Autodesk Fusion 360 part; units mm, degrees
note: some values were not read from the file. Set by a fixed rule: which face or edge a step refers to.
(part 3 of 12)
  spline S7 degree 5 poles (4.6371, -4.3427) (4.637, -4.3399) (4.6367, -4.3344) (4.6362, -4.326) (4.6355, -4.3149) (4.6346, -4.3011) (4.6336, -4.2873) (4.6327, -4.2735) (4.6316, -4.2598) (4.6306, -4.2461) (4.6295, -4.2324) (4.6283, -4.2188) (4.6271, -4.2052) (4.6259, -4.1917) (4.6246, -4.1782) (4.6233, -4.1647) (4.622, -4.1512) (4.6206, -4.1378) (4.6192, -4.1244) (4.6177, -4.1111) (4.6162, -4.0978) (4.6146, -4.0846) (4.6131, -4.0713) (4.6114, -4.0582) (4.6098, -4.045) (4.6081, -4.0319) (4.6063, -4.0188) (4.6045, -4.0058) (4.6027, -3.9928) (4.6009, -3.9799) (4.599, -3.967) (4.597, -3.9541) (4.5951, -3.9413) (4.5931, -3.9285) (4.591, -3.9157) (4.589, -3.903) (4.5868, -3.8904) (4.5847, -3.8778) (4.5825, -3.8652) (4.5803, -3.8526) (4.578, -3.8401) (4.5757, -3.8277) (4.5734, -3.8153) (4.5711, -3.8029) (4.5687, -3.7906) (4.5662, -3.7783) (4.5638, -3.766) (4.5613, -3.7538) (4.5587, -3.7417) (4.5562, -3.7296) (4.5536, -3.7175) (4.5509, -3.7055) (4.5483, -3.6935) (4.5456, -3.6816) (4.5429, -3.6697) (4.5401, -3.6578) (4.5373, -3.646) (4.5345, -3.6343) (4.5316, -3.6226) (4.5287, -3.6109) (4.5258, -3.5993) (4.5229, -3.5877) (4.5199, -3.5762) (4.5169, -3.5647) (4.5139, -3.5533) (4.5108, -3.5419) (4.5077, -3.5306) (4.5046, -3.5193) (4.5014, -3.508) (4.4983, -3.4969) (4.495, -3.4857) (4.4918, -3.4746) (4.4886, -3.4636) (4.4853, -3.4526) (4.4819, -3.4416) (4.4786, -3.4307) (4.4752, -3.4199) (4.4718, -3.4091) (4.4684, -3.3983) (4.465, -3.3876) (4.4615, -3.377) (4.458, -3.3664) (4.4545, -3.3558) (4.4509, -3.3453) (4.4474, -3.3349) (4.4438, -3.3245) (4.4402, -3.3141) (4.4365, -3.3039) (4.4329, -3.2936) (4.4292, -3.2834) (4.4255, -3.2733) (4.4218, -3.2632) (4.418, -3.2532) (4.4143, -3.2432) (4.4105, -3.2333) (4.4067, -3.2234) (4.4028, -3.2136) (4.399, -3.2038) (4.3951, -3.1941) (4.3912, -3.1845) (4.3873, -3.1749) (4.3834, -3.1653) (4.3795, -3.1558) (4.3755, -3.1464) (4.3715, -3.137) (4.3676, -3.1277) (4.3635, -3.1184) (4.3595, -3.1092) (4.3555, -3.1) (4.3514, -3.0909) (4.3474, -3.0819) (4.3433, -3.0729) (4.3392, -3.064) (4.3351, -3.0551) (4.331, -3.0463) (4.3268, -3.0375) (4.3227, -3.0288) (4.3185, -3.0202) (4.3143, -3.0116) (4.3102, -3.003) (4.306, -2.9946) (4.3018, -2.9862) (4.2975, -2.9778) (4.2933, -2.9695) (4.2891, -2.9613) (4.2848, -2.9531) (4.2806, -2.945) (4.2763, -2.9369) (4.2721, -2.9289) (4.2678, -2.921) (4.2635, -2.9131) (4.2592, -2.9053) (4.2549, -2.8975) (4.2507, -2.8898) (4.2464, -2.8822) (4.2421, -2.8746) (4.2377, -2.8671) (4.2334, -2.8596) (4.2291, -2.8522) (4.2248, -2.8449) (4.2205, -2.8376) (4.2162, -2.8304) (4.2119, -2.8233) (4.2075, -2.8162) (4.2032, -2.8092) (4.1989, -2.8022) (4.1946, -2.7953) (4.1903, -2.7885) (4.186, -2.7817) (4.1817, -2.775) (4.1774, -2.7684) (4.1731, -2.7618) (4.1688, -2.7553) (4.1645, -2.7488) (4.1602, -2.7424) (4.1559, -2.7361) (4.1516, -2.7298) (4.1474, -2.7236) (4.1431, -2.7175) (4.1389, -2.7115) (4.1346, -2.7055) (4.1304, -2.6995) (4.1262, -2.6936) (4.122, -2.6878) (4.1178, -2.6821) (4.1136, -2.6764) (4.1095, -2.6708) (4.1053, -2.6653) (4.1012, -2.6598) (4.097, -2.6544) (4.0929, -2.6491) (4.0888, -2.6438) (4.0848, -2.6386) (4.0807, -2.6335) (4.0767, -2.6284) (4.0726, -2.6234) (4.0686, -2.6184) (4.0647, -2.6136) (4.0607, -2.6088) (4.0568, -2.604) (4.0529, -2.5994) (4.049, -2.5948) (4.0451, -2.5902) (4.0413, -2.5858) (4.0375, -2.5814) (4.0337, -2.577) (4.0299, -2.5728) (4.0262, -2.5686) (4.0225, -2.5645) (4.0188, -2.5604) (4.0152, -2.5565) (4.0116, -2.5525) (4.008, -2.5487) (4.0044, -2.5449) (4.0009, -2.5412) (3.9975, -2.5376) (3.994, -2.534) (3.9906, -2.5305) (3.9873, -2.5271) (3.9839, -2.5237) (3.9807, -2.5205) (3.9774, -2.5172) (3.9742, -2.5141) (3.9711, -2.511) (3.968, -2.508) (3.9649, -2.5051) (3.9619, -2.5022) (3.9589, -2.4994) (3.956, -2.4967) (3.9531, -2.4941) (3.9503, -2.4915) (3.9475, -2.489) (3.9448, -2.4865) (3.9421, -2.4842) (3.9395, -2.4819) (3.937, -2.4797) (3.9345, -2.4775) (3.9321, -2.4754) (3.9297, -2.4734) (3.9274, -2.4715) (3.9251, -2.4696) (3.9229, -2.4678) (3.9208, -2.4661) (3.9188, -2.4644) (3.9168, -2.4629) (3.9149, -2.4613) (3.9131, -2.4599) (3.9113, -2.4585) (3.9096, -2.4572) (3.908, -2.456) (3.9065, -2.4549) (3.905, -2.4538) (3.9036, -2.4528) (3.9023, -2.4518) (3.9011, -2.451) (3.9, -2.4502) (3.899, -2.4495) (3.8981, -2.4488) (3.8972, -2.4482) (3.8965, -2.4477) (3.8958, -2.4473) (3.8954, -2.447) (3.8951, -2.4468) (3.8949, -2.4467) (3.8949, -2.4466) knots -1 -1 -1 -1 -1 -1 -0.99583333 -0.99166667 -0.9875 -0.98333333 -0.97916667 -0.975 -0.97083333 -0.96666667 -0.9625 -0.95833333 -0.95416667 -0.95 -0.94583333 -0.94166667 -0.9375 -0.93333333 -0.92916667 -0.925 -0.92083333 -0.91666667 -0.9125 -0.90833333 -0.90416667 -0.9 -0.89583333 -0.89166667 -0.8875 -0.88333333 -0.87916667 -0.875 -0.87083333 -0.86666667 -0.8625 -0.85833333 -0.85416667 -0.85 -0.84583333 -0.84166667 -0.8375 -0.83333333 -0.82916667 -0.825 -0.82083333 -0.81666667 -0.8125 -0.80833333 -0.80416667 -0.8 -0.79583333 -0.79166667 -0.7875 -0.78333333 -0.77916667 -0.775 -0.77083333 -0.76666667 -0.7625 -0.75833333 -0.75416667 -0.75 -0.74583333 -0.74166667 -0.7375 -0.73333333 -0.72916667 -0.725 -0.72083333 -0.71666667 -0.7125 -0.70833333 -0.70416667 -0.7 -0.69583333 -0.69166667 -0.6875 -0.68333333 -0.67916667 -0.675 -0.67083333 -0.66666667 -0.6625 -0.65833333 -0.65416667 -0.65 -0.64583333 -0.64166667 -0.6375 -0.63333333 -0.62916667 -0.625 -0.62083333 -0.61666667 -0.6125 -0.60833333 -0.60416667 -0.6 -0.59583333 -0.59166667 -0.5875 -0.58333333 -0.57916667 -0.575 -0.57083333 -0.56666667 -0.5625 -0.55833333 -0.55416667 -0.55 -0.54583333 -0.54166667 -0.5375 -0.53333333 -0.52916667 -0.525 -0.52083333 -0.51666667 -0.5125 -0.50833333 -0.50416667 -0.5 -0.49583333 -0.49166667 -0.4875 -0.48333333 -0.47916667 -0.475 -0.47083333 -0.46666667 -0.4625 -0.45833333 -0.45416667 -0.45 -0.44583333 -0.44166667 -0.4375 -0.43333333 -0.42916667 -0.425 -0.42083333 -0.41666667 -0.4125 -0.40833333 -0.40416667 -0.4 -0.39583333 -0.39166667 -0.3875 -0.38333333 -0.37916667 -0.375 -0.37083333 -0.36666667 -0.3625 -0.35833333 -0.35416667 -0.35 -0.34583333 -0.34166667 -0.3375 -0.33333333 -0.32916667 -0.325 -0.32083333 -0.31666667 -0.3125 -0.30833333 -0.30416667 -0.3 -0.29583333 -0.29166667 -0.2875 -0.28333333 -0.27916667 -0.275 -0.27083333 -0.26666667 -0.2625 -0.25833333 -0.25416667 -0.25 -0.24583333 -0.24166667 -0.2375 -0.23333333 -0.22916667 -0.225 -0.22083333 -0.21666667 -0.2125 -0.20833333 -0.20416667 -0.2 -0.19583333 -0.19166667 -0.1875 -0.18333333 -0.17916667 -0.175 -0.17083333 -0.16666667 -0.1625 -0.15833333 -0.15416667 -0.15 -0.14583333 -0.14166667 -0.1375 -0.13333333 -0.12916667 -0.125 -0.12083333 -0.11666667 -0.1125 -0.10833333 -0.10416667 -0.1 -0.09583333 -0.09166667 -0.0875 -0.08333333 -0.07916667 -0.075 -0.07083333 -0.06666667 -0.0625 -0.05833333 -0.05416667 -0.05 -0.04583333 -0.04166667 -0.0375 -0.03333333 -0.02916667 -0.025 -0.02083333 -0.01666667 -0.0125 -0.00833333 -0.00416667 0 0 0 0 0 0
  line L14 (3.8949, -2.4466) -> (3.8941, -2.4462)
  line L15 (3.8941, -2.4462) -> (3.1172, -1.9582)
  arc A8 (3.1172, -1.9582) -> (3.5889, -0.8196) centre (0, 0) ccw
  line L16 (3.5889, -0.8196) -> (4.4833, -1.0239)
  line L17 (4.4833, -1.0239) -> (4.4841, -1.024)
  spline S8 degree 5 poles (4.4841, -1.024) (4.4842, -1.0241) (4.4844, -1.0241) (4.4848, -1.0242) (4.4853, -1.0243) (4.486, -1.0244) (4.4869, -1.0246) (4.4879, -1.0248) (4.489, -1.025) (4.4903, -1.0252) (4.4916, -1.0254) (4.4931, -1.0257) (4.4947, -1.0259) (4.4963, -1.0262) (4.4981, -1.0264) (4.5, -1.0267) (4.502, -1.027) (4.5042, -1.0272) (4.5064, -1.0275) (4.5087, -1.0278) (4.5111, -1.0281) (4.5136, -1.0284) (4.5162, -1.0287) (4.5189, -1.0289) (4.5218, -1.0292) (4.5247, -1.0295) (4.5277, -1.0297) (4.5308, -1.03) (4.534, -1.0302) (4.5372, -1.0305) (4.5406, -1.0307) (4.5441, -1.0309) (4.5476, -1.0311) (4.5513, -1.0313) (4.555, -1.0315) (4.5588, -1.0317) (4.5627, -1.0319) (4.5667, -1.032) (4.5708, -1.0321) (4.575, -1.0322) (4.5792, -1.0323) (4.5835, -1.0324) (4.5879, -1.0325) (4.5924, -1.0325) (4.597, -1.0325) (4.6016, -1.0325) (4.6064, -1.0325) (4.6111, -1.0324) (4.616, -1.0324) (4.621, -1.0323) (4.626, -1.0322) (4.6311, -1.032) (4.6363, -1.0319) (4.6415, -1.0317) (4.6468, -1.0315) (4.6522, -1.0312) (4.6577, -1.031) (4.6632, -1.0307) (4.6688, -1.0303) (4.6745, -1.03) (4.6802, -1.0296) (4.686, -1.0292) (4.6919, -1.0288) (4.6978, -1.0283) (4.7038, -1.0278) (4.7099, -1.0272) (4.716, -1.0267) (4.7222, -1.0261) (4.7285, -1.0255) (4.7348, -1.0248) (4.7412, -1.0241) (4.7476, -1.0234) (4.7541, -1.0226) (4.7607, -1.0218) (4.7673, -1.021) (4.774, -1.0201) (4.7807, -1.0192) (4.7875, -1.0182) (4.7944, -1.0173) (4.8013, -1.0162) (4.8083, -1.0152) (4.8153, -1.0141) (4.8224, -1.013) (4.8295, -1.0118) (4.8367, -1.0106) (4.8439, -1.0093) (4.8512, -1.0081) (4.8585, -1.0067) (4.8659, -1.0054) (4.8734, -1.004) (4.8809, -1.0025) (4.8884, -1.001) (4.896, -0.9995) (4.9037, -0.9979) (4.9114, -0.9963) (4.9191, -0.9947) (4.9269, -0.993) (4.9347, -0.9912) (4.9426, -0.9894) (4.9505, -0.9876) (4.9585, -0.9858) (4.9665, -0.9838) (4.9746, -0.9819) (4.9827, -0.9799) (4.9908, -0.9778) (4.999, -0.9757) (5.0073, -0.9736) (5.0155, -0.9714) (5.0239, -0.9692) (5.0322, -0.9669) (5.0406, -0.9646) (5.0491, -0.9623) (5.0576, -0.9599) (5.0661, -0.9574) (5.0746, -0.9549) (5.0832, -0.9524) (5.0919, -0.9498) (5.1005, -0.9471) (5.1092, -0.9444) (5.118, -0.9417) (5.1268, -0.9389) (5.1356, -0.9361) (5.1444, -0.9332) (5.1533, -0.9303) (5.1623, -0.9273) (5.1712, -0.9243) (5.1802, -0.9212) (5.1892, -0.9181) (5.1983, -0.9149) (5.2074, -0.9117) (5.2165, -0.9084) (5.2256, -0.9051) (5.2348, -0.9017) (5.244, -0.8983) (5.2533, -0.8948) (5.2626, -0.8913) (5.2719, -0.8877) (5.2812, -0.8841) (5.2905, -0.8804) (5.2999, -0.8767) (5.3094, -0.8729) (5.3188, -0.8691) (5.3283, -0.8652) (5.3378, -0.8613) (5.3473, -0.8573) (5.3568, -0.8533) (5.3664, -0.8492) (5.376, -0.8451) (5.3856, -0.8409) (5.3953, -0.8367) (5.4049, -0.8324) (5.4146, -0.8281) (5.4244, -0.8237) (5.4341, -0.8192) (5.4439, -0.8147) (5.4537, -0.8102) (5.4635, -0.8056) (5.4733, -0.8009) (5.4831, -0.7962) (5.493, -0.7915) (5.5029, -0.7867) (5.5128, -0.7818) (5.5227, -0.7769) (5.5327, -0.7719) (5.5426, -0.7669) (5.5526, -0.7618) (5.5626, -0.7567) (5.5726, -0.7515) (5.5827, -0.7463) (5.5927, -0.741) (5.6028, -0.7356) (5.6129, -0.7302) (5.623, -0.7248) (5.6331, -0.7193) (5.6432, -0.7137) (5.6534, -0.7081) (5.6636, -0.7024) (5.6737, -0.6967) (5.6839, -0.6909) (5.6941, -0.6851) (5.7043, -0.6792) (5.7146, -0.6733) (5.7248, -0.6673) (5.7351, -0.6613) (5.7453, -0.6552) (5.7556, -0.649) (5.7659, -0.6428) (5.7762, -0.6365) (5.7865, -0.6302) (5.7968, -0.6239) (5.8071, -0.6174) (5.8175, -0.611) (5.8278, -0.6044) (5.8382, -0.5978) (5.8485, -0.5912) (5.8589, -0.5845) (5.8693, -0.5777) (5.8797, -0.5709) (5.8901, -0.5641) (5.9005, -0.5572) (5.9109, -0.5502) (5.9213, -0.5432) (5.9317, -0.5361) (5.9421, -0.529) (5.9525, -0.5218) (5.963, -0.5145) (5.9734, -0.5072) (5.9839, -0.4999) (5.9943, -0.4925) (6.0048, -0.485) (6.0152, -0.4775) (6.0257, -0.4699) (6.0361, -0.4623) (6.0466, -0.4546) (6.057, -0.4469) (6.0675, -0.4391) (6.078, -0.4313) (6.0884, -0.4234) (6.0989, -0.4154) (6.1094, -0.4074) (6.1199, -0.3993) (6.1303, -0.3912) (6.1408, -0.383) (6.1513, -0.3748) (6.1617, -0.3665) (6.1722, -0.3582) (6.1827, -0.3498) (6.1931, -0.3414) (6.2036, -0.3329) (6.2141, -0.3243) (6.2245, -0.3157) (6.235, -0.3071) (6.2454, -0.2983) (6.2559, -0.2896) (6.2663, -0.2807) (6.2768, -0.2719) (6.2872, -0.2629) (6.2976, -0.2539) (6.3081, -0.2449) (6.3185, -0.2358) (6.3289, -0.2267) (6.3372, -0.2193) (6.3435, -0.2137) (6.3476, -0.21) (6.3497, -0.2082) knots 0 0 0 0 0 0 0.00416667 0.00833333 0.0125 0.01666667 0.02083333 0.025 0.02916667 0.03333333 0.0375 0.04166667 0.04583333 0.05 0.05416667 0.05833333 0.0625 0.06666667 0.07083333 0.075 0.07916667 0.08333333 0.0875 0.09166667 0.09583333 0.1 0.10416667 0.10833333 0.1125 0.11666667 0.12083333 0.125 0.12916667 0.13333333 0.1375 0.14166667 0.14583333 0.15 0.15416667 0.15833333 0.1625 0.16666667 0.17083333 0.175 0.17916667 0.18333333 0.1875 0.19166667 0.19583333 0.2 0.20416667 0.20833333 0.2125 0.21666667 0.22083333 0.225 0.22916667 0.23333333 0.2375 0.24166667 0.24583333 0.25 0.25416667 0.25833333 0.2625 0.26666667 0.27083333 0.275 0.27916667 0.28333333 0.2875 0.29166667 0.29583333 0.3 0.30416667 0.30833333 0.3125 0.31666667 0.32083333 0.325 0.32916667 0.33333333 0.3375 0.34166667 0.34583333 0.35 0.35416667 0.35833333 0.3625 0.36666667 0.37083333 0.375 0.37916667 0.38333333 0.3875 0.39166667 0.39583333 0.4 0.40416667 0.40833333 0.4125 0.41666667 0.42083333 0.425 0.42916667 0.43333333 0.4375 0.44166667 0.44583333 0.45 0.45416667 0.45833333 0.4625 0.46666667 0.47083333 0.475 0.47916667 0.48333333 0.4875 0.49166667 0.49583333 0.5 0.50416667 0.50833333 0.5125 0.51666667 0.52083333 0.525 0.52916667 0.53333333 0.5375 0.54166667 0.54583333 0.55 0.55416667 0.55833333 0.5625 0.56666667 0.57083333 0.575 0.57916667 0.58333333 0.5875 0.59166667 0.59583333 0.6 0.60416667 0.60833333 0.6125 0.61666667 0.62083333 0.625 0.62916667 0.63333333 0.6375 0.64166667 0.64583333 0.65 0.65416667 0.65833333 0.6625 0.66666667 0.67083333 0.675 0.67916667 0.68333333 0.6875 0.69166667 0.69583333 0.7 0.70416667 0.70833333 0.7125 0.71666667 0.72083333 0.725 0.72916667 0.73333333 0.7375 0.74166667 0.74583333 0.75 0.75416667 0.75833333 0.7625 0.76666667 0.77083333 0.775 0.77916667 0.78333333 0.7875 0.79166667 0.79583333 0.8 0.80416667 0.80833333 0.8125 0.81666667 0.82083333 0.825 0.82916667 0.83333333 0.8375 0.84166667 0.84583333 0.85 0.85416667 0.85833333 0.8625 0.86666667 0.87083333 0.875 0.87916667 0.88333333 0.8875 0.89166667 0.89583333 0.9 0.90416667 0.90833333 0.9125 0.91666667 0.92083333 0.925 0.92916667 0.93333333 0.9375 0.94166667 0.94583333 0.95 0.95416667 0.95833333 0.9625 0.96666667 0.97083333 0.975 0.97916667 0.98333333 0.9875 0.99166667 0.99583333 1 1 1 1 1 1
  arc A9 (6.3497, -0.2082) -> (6.3497, 0.2082) centre (0, 0) ccw
  spline S9 degree 5 poles (6.3497, 0.2082) (6.3476, 0.21) (6.3435, 0.2137) (6.3372, 0.2193) (6.3289, 0.2267) (6.3185, 0.2358) (6.3081, 0.2449) (6.2976, 0.2539) (6.2872, 0.2629) (6.2768, 0.2719) (6.2663, 0.2807) (6.2559, 0.2896) (6.2454, 0.2983) (6.235, 0.3071) (6.2245, 0.3157) (6.2141, 0.3243) (6.2036, 0.3329) (6.1931, 0.3414) (6.1827, 0.3498) (6.1722, 0.3582) (6.1617, 0.3665) (6.1513, 0.3748) (6.1408, 0.383) (6.1303, 0.3912) (6.1199, 0.3993) (6.1094, 0.4074) (6.0989, 0.4154) (6.0884, 0.4234) (6.078, 0.4313) (6.0675, 0.4391) (6.057, 0.4469) (6.0466, 0.4546) (6.0361, 0.4623) (6.0257, 0.4699) (6.0152, 0.4775) (6.0048, 0.485) (5.9943, 0.4925) (5.9839, 0.4999) (5.9734, 0.5072) (5.963, 0.5145) (5.9525, 0.5218) (5.9421, 0.529) (5.9317, 0.5361) (5.9213, 0.5432) (5.9109, 0.5502) (5.9005, 0.5572) (5.8901, 0.5641) (5.8797, 0.5709) (5.8693, 0.5777) (5.8589, 0.5845) (5.8485, 0.5912) (5.8382, 0.5978) (5.8278, 0.6044) (5.8175, 0.611) (5.8071, 0.6174) (5.7968, 0.6239) (5.7865, 0.6302) (5.7762, 0.6365) (5.7659, 0.6428) (5.7556, 0.649) (5.7453, 0.6552) (5.7351, 0.6613) (5.7248, 0.6673) (5.7146, 0.6733) (5.7043, 0.6792) (5.6941, 0.6851) (5.6839, 0.6909) (5.6737, 0.6967) (5.6636, 0.7024) (5.6534, 0.7081) (5.6432, 0.7137) (5.6331, 0.7193) (5.623, 0.7248) (5.6129, 0.7302) (5.6028, 0.7356) (5.5927, 0.741) (5.5827, 0.7463) (5.5726, 0.7515) (5.5626, 0.7567) (5.5526, 0.7618) (5.5426, 0.7669) (5.5327, 0.7719) (5.5227, 0.7769) (5.5128, 0.7818) (5.5029, 0.7867) (5.493, 0.7915) (5.4831, 0.7962) (5.4733, 0.8009) (5.4635, 0.8056) (5.4537, 0.8102) (5.4439, 0.8147) (5.4341, 0.8192) (5.4244, 0.8237) (5.4146, 0.8281) (5.4049, 0.8324) (5.3953, 0.8367) (5.3856, 0.8409) (5.376, 0.8451) (5.3664, 0.8492) (5.3568, 0.8533) (5.3473, 0.8573) (5.3378, 0.8613) (5.3283, 0.8652) (5.3188, 0.8691) (5.3094, 0.8729) (5.2999, 0.8767) (5.2905, 0.8804) (5.2812, 0.8841) (5.2719, 0.8877) (5.2626, 0.8913) (5.2533, 0.8948) (5.244, 0.8983) (5.2348, 0.9017) (5.2256, 0.9051) (5.2165, 0.9084) (5.2074, 0.9117) (5.1983, 0.9149) (5.1892, 0.9181) (5.1802, 0.9212) (5.1712, 0.9243) (5.1623, 0.9273) (5.1533, 0.9303) (5.1444, 0.9332) (5.1356, 0.9361) (5.1268, 0.9389) (5.118, 0.9417) (5.1092, 0.9444) (5.1005, 0.9471) (5.0919, 0.9498) (5.0832, 0.9524) (5.0746, 0.9549) (5.0661, 0.9574) (5.0576, 0.9599) (5.0491, 0.9623) (5.0406, 0.9646) (5.0322, 0.9669) (5.0239, 0.9692) (5.0155, 0.9714) (5.0073, 0.9736) (4.999, 0.9757) (4.9908, 0.9778) (4.9827, 0.9799) (4.9746, 0.9819) (4.9665, 0.9838) (4.9585, 0.9858) (4.9505, 0.9876) (4.9426, 0.9894) (4.9347, 0.9912) (4.9269, 0.993) (4.9191, 0.9947) (4.9114, 0.9963) (4.9037, 0.9979) (4.896, 0.9995) (4.8884, 1.001) (4.8809, 1.0025) (4.8734, 1.004) (4.8659, 1.0054) (4.8585, 1.0067) (4.8512, 1.0081) (4.8439, 1.0093) (4.8367, 1.0106) (4.8295, 1.0118) (4.8224, 1.013) (4.8153, 1.0141) (4.8083, 1.0152) (4.8013, 1.0162) (4.7944, 1.0173) (4.7875, 1.0182) (4.7807, 1.0192) (4.774, 1.0201) (4.7673, 1.021) (4.7607, 1.0218) (4.7541, 1.0226) (4.7476, 1.0234) (4.7412, 1.0241) (4.7348, 1.0248) (4.7285, 1.0255) (4.7222, 1.0261) (4.716, 1.0267) (4.7099, 1.0272) (4.7038, 1.0278) (4.6978, 1.0283) (4.6919, 1.0288) (4.686, 1.0292) (4.6802, 1.0296) (4.6745, 1.03) (4.6688, 1.0303) (4.6632, 1.0307) (4.6577, 1.031) (4.6522, 1.0312) (4.6468, 1.0315) (4.6415, 1.0317) (4.6363, 1.0319) (4.6311, 1.032) (4.626, 1.0322) (4.621, 1.0323) (4.616, 1.0324) (4.6111, 1.0324) (4.6064, 1.0325) (4.6016, 1.0325) (4.597, 1.0325) (4.5924, 1.0325) (4.5879, 1.0325) (4.5835, 1.0324) (4.5792, 1.0323) (4.575, 1.0322) (4.5708, 1.0321) (4.5667, 1.032) (4.5627, 1.0319) (4.5588, 1.0317) (4.555, 1.0315) (4.5513, 1.0313) (4.5476, 1.0311) (4.5441, 1.0309) (4.5406, 1.0307) (4.5372, 1.0305) (4.534, 1.0302) (4.5308, 1.03) (4.5277, 1.0297) (4.5247, 1.0295) (4.5218, 1.0292) (4.5189, 1.0289) (4.5162, 1.0287) (4.5136, 1.0284) (4.5111, 1.0281) (4.5087, 1.0278) (4.5064, 1.0275) (4.5042, 1.0272) (4.502, 1.027) (4.5, 1.0267) (4.4981, 1.0264) (4.4963, 1.0262) (4.4947, 1.0259) (4.4931, 1.0257) (4.4916, 1.0254) (4.4903, 1.0252) (4.489, 1.025) (4.4879, 1.0248) (4.4869, 1.0246) (4.486, 1.0244) (4.4853, 1.0243) (4.4848, 1.0242) (4.4844, 1.0241) (4.4842, 1.0241) (4.4841, 1.024) knots -1 -1 -1 -1 -1 -1 -0.99583333 -0.99166667 -0.9875 -0.98333333 -0.97916667 -0.975 -0.97083333 -0.96666667 -0.9625 -0.95833333 -0.95416667 -0.95 -0.94583333 -0.94166667 -0.9375 -0.93333333 -0.92916667 -0.925 -0.92083333 -0.91666667 -0.9125 -0.90833333 -0.90416667 -0.9 -0.89583333 -0.89166667 -0.8875 -0.88333333 -0.87916667 -0.875 -0.87083333 -0.86666667 -0.8625 -0.85833333 -0.85416667 -0.85 -0.84583333 -0.84166667 -0.8375 -0.83333333 -0.82916667 -0.825 -0.82083333 -0.81666667 -0.8125 -0.80833333 -0.80416667 -0.8 -0.79583333 -0.79166667 -0.7875 -0.78333333 -0.77916667 -0.775 -0.77083333 -0.76666667 -0.7625 -0.75833333 -0.75416667 -0.75 -0.74583333 -0.74166667 -0.7375 -0.73333333 -0.72916667 -0.725 -0.72083333 -0.71666667 -0.7125 -0.70833333 -0.70416667 -0.7 -0.69583333 -0.69166667 -0.6875 -0.68333333 -0.67916667 -0.675 -0.67083333 -0.66666667 -0.6625 -0.65833333 -0.65416667 -0.65 -0.64583333 -0.64166667 -0.6375 -0.63333333 -0.62916667 -0.625 -0.62083333 -0.61666667 -0.6125 -0.60833333 -0.60416667 -0.6 -0.59583333 -0.59166667 -0.5875 -0.58333333 -0.57916667 -0.575 -0.57083333 -0.56666667 -0.5625 -0.55833333 -0.55416667 -0.55 -0.54583333 -0.54166667 -0.5375 -0.53333333 -0.52916667 -0.525 -0.52083333 -0.51666667 -0.5125 -0.50833333 -0.50416667 -0.5 -0.49583333 -0.49166667 -0.4875 -0.48333333 -0.47916667 -0.475 -0.47083333 -0.46666667 -0.4625 -0.45833333 -0.45416667 -0.45 -0.44583333 -0.44166667 -0.4375 -0.43333333 -0.42916667 -0.425 -0.42083333 -0.41666667 -0.4125 -0.40833333 -0.40416667 -0.4 -0.39583333 -0.39166667 -0.3875 -0.38333333 -0.37916667 -0.375 -0.37083333 -0.36666667 -0.3625 -0.35833333 -0.35416667 -0.35 -0.34583333 -0.34166667 -0.3375 -0.33333333 -0.32916667 -0.325 -0.32083333 -0.31666667 -0.3125 -0.30833333 -0.30416667 -0.3 -0.29583333 -0.29166667 -0.2875 -0.28333333 -0.27916667 -0.275 -0.27083333 -0.26666667 -0.2625 -0.25833333 -0.25416667 -0.25 -0.24583333 -0.24166667 -0.2375 -0.23333333 -0.22916667 -0.225 -0.22083333 -0.21666667 -0.2125 -0.20833333 -0.20416667 -0.2 -0.19583333 -0.19166667 -0.1875 -0.18333333 -0.17916667 -0.175 -0.17083333 -0.16666667 -0.1625 -0.15833333 -0.15416667 -0.15 -0.14583333 -0.14166667 -0.1375 -0.13333333 -0.12916667 -0.125 -0.12083333 -0.11666667 -0.1125 -0.10833333 -0.10416667 -0.1 -0.09583333 -0.09166667 -0.0875 -0.08333333 -0.07916667 -0.075 -0.07083333 -0.06666667 -0.0625 -0.05833333 -0.05416667 -0.05 -0.04583333 -0.04166667 -0.0375 -0.03333333 -0.02916667 -0.025 -0.02083333 -0.01666667 -0.0125 -0.00833333 -0.00416667 0 0 0 0 0 0
  line L18 (4.4841, 1.024) -> (4.4833, 1.0239)
  line L19 (4.4833, 1.0239) -> (3.5889, 0.8196)
  arc A10 (3.5889, 0.8196) -> (3.1172, 1.9582) centre (0, 0) ccw
  line L20 (3.1172, 1.9582) -> (3.8941, 2.4462)
  line L21 (3.8941, 2.4462) -> (3.8949, 2.4466)
  spline S10 degree 5 poles (3.8949, 2.4466) (3.8949, 2.4467) (3.8951, 2.4468) (3.8954, 2.447) (3.8958, 2.4473) (3.8965, 2.4477) (3.8972, 2.4482) (3.8981, 2.4488) (3.899, 2.4495) (3.9, 2.4502) (3.9011, 2.451) (3.9023, 2.4518) (3.9036, 2.4528) (3.905, 2.4538) (3.9065, 2.4549) (3.908, 2.456) (3.9096, 2.4572) (3.9113, 2.4585) (3.9131, 2.4599) (3.9149, 2.4613) (3.9168, 2.4629) (3.9188, 2.4644) (3.9208, 2.4661) (3.9229, 2.4678) (3.9251, 2.4696) (3.9274, 2.4715) (3.9297, 2.4734) (3.9321, 2.4754) (3.9345, 2.4775) (3.937, 2.4797) (3.9395, 2.4819) (3.9421, 2.4842) (3.9448, 2.4865) (3.9475, 2.489) (3.9503, 2.4915) (3.9531, 2.4941) (3.956, 2.4967) (3.9589, 2.4994) (3.9619, 2.5022) (3.9649, 2.5051) (3.968, 2.508) (3.9711, 2.511) (3.9742, 2.5141) (3.9774, 2.5172) (3.9807, 2.5205) (3.9839, 2.5237) (3.9873, 2.5271) (3.9906, 2.5305) (3.994, 2.534) (3.9975, 2.5376) (4.0009, 2.5412) (4.0044, 2.5449) (4.008, 2.5487) (4.0116, 2.5525) (4.0152, 2.5565) (4.0188, 2.5604) (4.0225, 2.5645) (4.0262, 2.5686) (4.0299, 2.5728) (4.0337, 2.577) (4.0375, 2.5814) (4.0413, 2.5858) (4.0451, 2.5902) (4.049, 2.5948) (4.0529, 2.5994) (4.0568, 2.604) (4.0607, 2.6088) (4.0647, 2.6136) (4.0686, 2.6184) (4.0726, 2.6234) (4.0767, 2.6284) (4.0807, 2.6335) (4.0848, 2.6386) (4.0888, 2.6438) (4.0929, 2.6491) (4.097, 2.6544) (4.1012, 2.6598) (4.1053, 2.6653) (4.1095, 2.6708) (4.1136, 2.6764) (4.1178, 2.6821) (4.122, 2.6878) (4.1262, 2.6936) (4.1304, 2.6995) (4.1346, 2.7055) (4.1389, 2.7115) (4.1431, 2.7175) (4.1474, 2.7236) (4.1516, 2.7298) (4.1559, 2.7361) (4.1602, 2.7424) (4.1645, 2.7488) (4.1688, 2.7553) (4.1731, 2.7618) (4.1774, 2.7684) (4.1817, 2.775) (4.186, 2.7817) (4.1903, 2.7885) (4.1946, 2.7953) (4.1989, 2.8022) (4.2032, 2.8092) (4.2075, 2.8162) (4.2119, 2.8233) (4.2162, 2.8304) (4.2205, 2.8376) (4.2248, 2.8449) (4.2291, 2.8522) (4.2334, 2.8596) (4.2377, 2.8671) (4.2421, 2.8746) (4.2464, 2.8822) (4.2507, 2.8898) (4.2549, 2.8975) (4.2592, 2.9053) (4.2635, 2.9131) (4.2678, 2.921) (4.2721, 2.9289) (4.2763, 2.9369) (4.2806, 2.945) (4.2848, 2.9531) (4.2891, 2.9613) (4.2933, 2.9695) (4.2975, 2.9778) (4.3018, 2.9862) (4.306, 2.9946) (4.3102, 3.003) (4.3143, 3.0116) (4.3185, 3.0202) (4.3227, 3.0288) (4.3268, 3.0375) (4.331, 3.0463) (4.3351, 3.0551) (4.3392, 3.064) (4.3433, 3.0729) (4.3474, 3.0819) (4.3514, 3.0909) (4.3555, 3.1) (4.3595, 3.1092) (4.3635, 3.1184) (4.3676, 3.1277) (4.3715, 3.137) (4.3755, 3.1464) (4.3795, 3.1558) (4.3834, 3.1653) (4.3873, 3.1749) (4.3912, 3.1845) (4.3951, 3.1941) (4.399, 3.2038) (4.4028, 3.2136) (4.4067, 3.2234) (4.4105, 3.2333) (4.4143, 3.2432) (4.418, 3.2532) (4.4218, 3.2632) (4.4255, 3.2733) (4.4292, 3.2834) (4.4329, 3.2936) (4.4365, 3.3039) (4.4402, 3.3141) (4.4438, 3.3245) (4.4474, 3.3349) (4.4509, 3.3453) (4.4545, 3.3558) (4.458, 3.3664) (4.4615, 3.377) (4.465, 3.3876) (4.4684, 3.3983) (4.4718, 3.4091) (4.4752, 3.4199) (4.4786, 3.4307) (4.4819, 3.4416) (4.4853, 3.4526) (4.4886, 3.4636) (4.4918, 3.4746) (4.495, 3.4857) (4.4983, 3.4969) (4.5014, 3.508) (4.5046, 3.5193) (4.5077, 3.5306) (4.5108, 3.5419) (4.5139, 3.5533) (4.5169, 3.5647) (4.5199, 3.5762) (4.5229, 3.5877) (4.5258, 3.5993) (4.5287, 3.6109) (4.5316, 3.6226) (4.5345, 3.6343) (4.5373, 3.646) (4.5401, 3.6578) (4.5429, 3.6697) (4.5456, 3.6816) (4.5483, 3.6935) (4.5509, 3.7055) (4.5536, 3.7175) (4.5562, 3.7296) (4.5587, 3.7417) (4.5613, 3.7538) (4.5638, 3.766) (4.5662, 3.7783) (4.5687, 3.7906) (4.5711, 3.8029) (4.5734, 3.8153) (4.5757, 3.8277) (4.578, 3.8401) (4.5803, 3.8526) (4.5825, 3.8652) (4.5847, 3.8778) (4.5868, 3.8904) (4.589, 3.903) (4.591, 3.9157) (4.5931, 3.9285) (4.5951, 3.9413) (4.597, 3.9541) (4.599, 3.967) (4.6009, 3.9799) (4.6027, 3.9928) (4.6045, 4.0058) (4.6063, 4.0188) (4.6081, 4.0319) (4.6098, 4.045) (4.6114, 4.0582) (4.6131, 4.0713) (4.6146, 4.0846) (4.6162, 4.0978) (4.6177, 4.1111) (4.6192, 4.1244) (4.6206, 4.1378) (4.622, 4.1512) (4.6233, 4.1647) (4.6246, 4.1782) (4.6259, 4.1917) (4.6271, 4.2052) (4.6283, 4.2188) (4.6295, 4.2324) (4.6306, 4.2461) (4.6316, 4.2598) (4.6327, 4.2735) (4.6336, 4.2873) (4.6346, 4.3011) (4.6355, 4.3149) (4.6362, 4.326) (4.6367, 4.3344) (4.637, 4.3399) (4.6371, 4.3427) knots 0 0 0 0 0 0 0.00416667 0.00833333 0.0125 0.01666667 0.02083333 0.025 0.02916667 0.03333333 0.0375 0.04166667 0.04583333 0.05 0.05416667 0.05833333 0.0625 0.06666667 0.07083333 0.075 0.07916667 0.08333333 0.0875 0.09166667 0.09583333 0.1 0.10416667 0.10833333 0.1125 0.11666667 0.12083333 0.125 0.12916667 0.13333333 0.1375 0.14166667 0.14583333 0.15 0.15416667 0.15833333 0.1625 0.16666667 0.17083333 0.175 0.17916667 0.18333333 0.1875 0.19166667 0.19583333 0.2 0.20416667 0.20833333 0.2125 0.21666667 0.22083333 0.225 0.22916667 0.23333333 0.2375 0.24166667 0.24583333 0.25 0.25416667 0.25833333 0.2625 0.26666667 0.27083333 0.275 0.27916667 0.28333333 0.2875 0.29166667 0.29583333 0.3 0.30416667 0.30833333 0.3125 0.31666667 0.32083333 0.325 0.32916667 0.33333333 0.3375 0.34166667 0.34583333 0.35 0.35416667 0.35833333 0.3625 0.36666667 0.37083333 0.375 0.37916667 0.38333333 0.3875 0.39166667 0.39583333 0.4 0.40416667 0.40833333 0.4125 0.41666667 0.42083333 0.425 0.42916667 0.43333333 0.4375 0.44166667 0.44583333 0.45 0.45416667 0.45833333 0.4625 0.46666667 0.47083333 0.475 0.47916667 0.48333333 0.4875 0.49166667 0.49583333 0.5 0.50416667 0.50833333 0.5125 0.51666667 0.52083333 0.525 0.52916667 0.53333333 0.5375 0.54166667 0.54583333 0.55 0.55416667 0.55833333 0.5625 0.56666667 0.57083333 0.575 0.57916667 0.58333333 0.5875 0.59166667 0.59583333 0.6 0.60416667 0.60833333 0.6125 0.61666667 0.62083333 0.625 0.62916667 0.63333333 0.6375 0.64166667 0.64583333 0.65 0.65416667 0.65833333 0.6625 0.66666667 0.67083333 0.675 0.67916667 0.68333333 0.6875 0.69166667 0.69583333 0.7 0.70416667 0.70833333 0.7125 0.71666667 0.72083333 0.725 0.72916667 0.73333333 0.7375 0.74166667 0.74583333 0.75 0.75416667 0.75833333 0.7625 0.76666667 0.77083333 0.775 0.77916667 0.78333333 0.7875 0.79166667 0.79583333 0.8 0.80416667 0.80833333 0.8125 0.81666667 0.82083333 0.825 0.82916667 0.83333333 0.8375 0.84166667 0.84583333 0.85 0.85416667 0.85833333 0.8625 0.86666667 0.87083333 0.875 0.87916667 0.88333333 0.8875 0.89166667 0.89583333 0.9 0.90416667 0.90833333 0.9125 0.91666667 0.92083333 0.925 0.92916667 0.93333333 0.9375 0.94166667 0.94583333 0.95 0.95416667 0.95833333 0.9625 0.96666667 0.97083333 0.975 0.97916667 0.98333333 0.9875 0.99166667 0.99583333 1 1 1 1 1 1
  arc A11 (4.6371, 4.3427) -> (4.3427, 4.6371) centre (0, 0) ccw
  spline S11 degree 5 poles (4.3427, 4.6371) (4.3399, 4.637) (4.3344, 4.6367) (4.326, 4.6362) (4.3149, 4.6355) (4.3011, 4.6346) (4.2873, 4.6336) (4.2735, 4.6327) (4.2598, 4.6316) (4.2461, 4.6306) (4.2324, 4.6295) (4.2188, 4.6283) (4.2052, 4.6271) (4.1917, 4.6259) (4.1782, 4.6246) (4.1647, 4.6233) (4.1512, 4.622) (4.1378, 4.6206) (4.1244, 4.6192) (4.1111, 4.6177) (4.0978, 4.6162) (4.0846, 4.6146) (4.0713, 4.6131) (4.0582, 4.6114) (4.045, 4.6098) (4.0319, 4.6081) (4.0188, 4.6063) (4.0058, 4.6045) (3.9928, 4.6027) (3.9799, 4.6009) (3.967, 4.599) (3.9541, 4.597) (3.9413, 4.5951) (3.9285, 4.5931) (3.9157, 4.591) (3.903, 4.589) (3.8904, 4.5868) (3.8778, 4.5847) (3.8652, 4.5825) (3.8526, 4.5803) (3.8401, 4.578) (3.8277, 4.5757) (3.8153, 4.5734) (3.8029, 4.5711) (3.7906, 4.5687) (3.7783, 4.5662) (3.766, 4.5638) (3.7538, 4.5613) (3.7417, 4.5587) (3.7296, 4.5562) (3.7175, 4.5536) (3.7055, 4.5509) (3.6935, 4.5483) (3.6816, 4.5456) (3.6697, 4.5429) (3.6578, 4.5401) (3.646, 4.5373) (3.6343, 4.5345) (3.6226, 4.5316) (3.6109, 4.5287) (3.5993, 4.5258) (3.5877, 4.5229) (3.5762, 4.5199) (3.5647, 4.5169) (3.5533, 4.5139) (3.5419, 4.5108) (3.5306, 4.5077) (3.5193, 4.5046) (3.508, 4.5014) (3.4969, 4.4983) (3.4857, 4.495) (3.4746, 4.4918) (3.4636, 4.4886) (3.4526, 4.4853) (3.4416, 4.4819) (3.4307, 4.4786) (3.4199, 4.4752) (3.4091, 4.4718) (3.3983, 4.4684) (3.3876, 4.465) (3.377, 4.4615) (3.3664, 4.458) (3.3558, 4.4545) (3.3453, 4.4509) (3.3349, 4.4474) (3.3245, 4.4438) (3.3141, 4.4402) (3.3039, 4.4365) (3.2936, 4.4329) (3.2834, 4.4292) (3.2733, 4.4255) (3.2632, 4.4218) (3.2532, 4.418) (3.2432, 4.4143) (3.2333, 4.4105) (3.2234, 4.4067) (3.2136, 4.4028) (3.2038, 4.399) (3.1941, 4.3951) (3.1845, 4.3912) (3.1749, 4.3873) (3.1653, 4.3834) (3.1558, 4.3795) (3.1464, 4.3755) (3.137, 4.3715) (3.1277, 4.3676) (3.1184, 4.3635) (3.1092, 4.3595) (3.1, 4.3555) (3.0909, 4.3514) (3.0819, 4.3474) (3.0729, 4.3433) (3.064, 4.3392) (3.0551, 4.3351) (3.0463, 4.331) (3.0375, 4.3268) (3.0288, 4.3227) (3.0202, 4.3185) (3.0116, 4.3143) (3.003, 4.3102) (2.9946, 4.306) (2.9862, 4.3018) (2.9778, 4.2975) (2.9695, 4.2933) (2.9613, 4.2891) (2.9531, 4.2848) (2.945, 4.2806) (2.9369, 4.2763) (2.9289, 4.2721) (2.921, 4.2678) (2.9131, 4.2635) (2.9053, 4.2592) (2.8975, 4.2549) (2.8898, 4.2507) (2.8822, 4.2464) (2.8746, 4.2421) (2.8671, 4.2377) (2.8596, 4.2334) (2.8522, 4.2291) (2.8449, 4.2248) (2.8376, 4.2205) (2.8304, 4.2162) (2.8233, 4.2119) (2.8162, 4.2075) (2.8092, 4.2032) (2.8022, 4.1989) (2.7953, 4.1946) (2.7885, 4.1903) (2.7817, 4.186) (2.775, 4.1817) (2.7684, 4.1774) (2.7618, 4.1731) (2.7553, 4.1688) (2.7488, 4.1645) (2.7424, 4.1602) (2.7361, 4.1559) (2.7298, 4.1516) (2.7236, 4.1474) (2.7175, 4.1431) (2.7115, 4.1389) (2.7055, 4.1346) (2.6995, 4.1304) (2.6936, 4.1262) (2.6878, 4.122) (2.6821, 4.1178) (2.6764, 4.1136) (2.6708, 4.1095) (2.6653, 4.1053) (2.6598, 4.1012) (2.6544, 4.097) (2.6491, 4.0929) (2.6438, 4.0888) (2.6386, 4.0848) (2.6335, 4.0807) (2.6284, 4.0767) (2.6234, 4.0726) (2.6184, 4.0686) (2.6136, 4.0647) (2.6088, 4.0607) (2.604, 4.0568) (2.5994, 4.0529) (2.5948, 4.049) (2.5902, 4.0451) (2.5858, 4.0413) (2.5814, 4.0375) (2.577, 4.0337) (2.5728, 4.0299) (2.5686, 4.0262) (2.5645, 4.0225) (2.5604, 4.0188) (2.5565, 4.0152) (2.5525, 4.0116) (2.5487, 4.008) (2.5449, 4.0044) (2.5412, 4.0009) (2.5376, 3.9975) (2.534, 3.994) (2.5305, 3.9906) (2.5271, 3.9873) (2.5237, 3.9839) (2.5205, 3.9807) (2.5172, 3.9774) (2.5141, 3.9742) (2.511, 3.9711) (2.508, 3.968) (2.5051, 3.9649) (2.5022, 3.9619) (2.4994, 3.9589) (2.4967, 3.956) (2.4941, 3.9531) (2.4915, 3.9503) (2.489, 3.9475) (2.4865, 3.9448) (2.4842, 3.9421) (2.4819, 3.9395) (2.4797, 3.937) (2.4775, 3.9345) (2.4754, 3.9321) (2.4734, 3.9297) (2.4715, 3.9274) (2.4696, 3.9251) (2.4678, 3.9229) (2.4661, 3.9208) (2.4644, 3.9188) (2.4629, 3.9168) (2.4613, 3.9149) (2.4599, 3.9131) (2.4585, 3.9113) (2.4572, 3.9096) (2.456, 3.908) (2.4549, 3.9065) (2.4538, 3.905) (2.4528, 3.9036) (2.4518, 3.9023) (2.451, 3.9011) (2.4502, 3.9) (2.4495, 3.899) (2.4488, 3.8981) (2.4482, 3.8972) (2.4477, 3.8965) (2.4473, 3.8958) (2.447, 3.8954) (2.4468, 3.8951) (2.4467, 3.8949) (2.4466, 3.8949) knots -1 -1 -1 -1 -1 -1 -0.99583333 -0.99166667 -0.9875 -0.98333333 -0.97916667 -0.975 -0.97083333 -0.96666667 -0.9625 -0.95833333 -0.95416667 -0.95 -0.94583333 -0.94166667 -0.9375 -0.93333333 -0.92916667 -0.925 -0.92083333 -0.91666667 -0.9125 -0.90833333 -0.90416667 -0.9 -0.89583333 -0.89166667 -0.8875 -0.88333333 -0.87916667 -0.875 -0.87083333 -0.86666667 -0.8625 -0.85833333 -0.85416667 -0.85 -0.84583333 -0.84166667 -0.8375 -0.83333333 -0.82916667 -0.825 -0.82083333 -0.81666667 -0.8125 -0.80833333 -0.80416667 -0.8 -0.79583333 -0.79166667 -0.7875 -0.78333333 -0.77916667 -0.775 -0.77083333 -0.76666667 -0.7625 -0.75833333 -0.75416667 -0.75 -0.74583333 -0.74166667 -0.7375 -0.73333333 -0.72916667 -0.725 -0.72083333 -0.71666667 -0.7125 -0.70833333 -0.70416667 -0.7 -0.69583333 -0.69166667 -0.6875 -0.68333333 -0.67916667 -0.675 -0.67083333 -0.66666667 -0.6625 -0.65833333 -0.65416667 -0.65 -0.64583333 -0.64166667 -0.6375 -0.63333333 -0.62916667 -0.625 -0.62083333 -0.61666667 -0.6125 -0.60833333 -0.60416667 -0.6 -0.59583333 -0.59166667 -0.5875 -0.58333333 -0.57916667 -0.575 -0.57083333 -0.56666667 -0.5625 -0.55833333 -0.55416667 -0.55 -0.54583333 -0.54166667 -0.5375 -0.53333333 -0.52916667 -0.525 -0.52083333 -0.51666667 -0.5125 -0.50833333 -0.50416667 -0.5 -0.49583333 -0.49166667 -0.4875 -0.48333333 -0.47916667 -0.475 -0.47083333 -0.46666667 -0.4625 -0.45833333 -0.45416667 -0.45 -0.44583333 -0.44166667 -0.4375 -0.43333333 -0.42916667 -0.425 -0.42083333 -0.41666667 -0.4125 -0.40833333 -0.40416667 -0.4 -0.39583333 -0.39166667 -0.3875 -0.38333333 -0.37916667 -0.375 -0.37083333 -0.36666667 -0.3625 -0.35833333 -0.35416667 -0.35 -0.34583333 -0.34166667 -0.3375 -0.33333333 -0.32916667 -0.325 -0.32083333 -0.31666667 -0.3125 -0.30833333 -0.30416667 -0.3 -0.29583333 -0.29166667 -0.2875 -0.28333333 -0.27916667 -0.275 -0.27083333 -0.26666667 -0.2625 -0.25833333 -0.25416667 -0.25 -0.24583333 -0.24166667 -0.2375 -0.23333333 -0.22916667 -0.225 -0.22083333 -0.21666667 -0.2125 -0.20833333 -0.20416667 -0.2 -0.19583333 -0.19166667 -0.1875 -0.18333333 -0.17916667 -0.175 -0.17083333 -0.16666667 -0.1625 -0.15833333 -0.15416667 -0.15 -0.14583333 -0.14166667 -0.1375 -0.13333333 -0.12916667 -0.125 -0.12083333 -0.11666667 -0.1125 -0.10833333 -0.10416667 -0.1 -0.09583333 -0.09166667 -0.0875 -0.08333333 -0.07916667 -0.075 -0.07083333 -0.06666667 -0.0625 -0.05833333 -0.05416667 -0.05 -0.04583333 -0.04166667 -0.0375 -0.03333333 -0.02916667 -0.025 -0.02083333 -0.01666667 -0.0125 -0.00833333 -0.00416667 0 0 0 0 0 0
  line L22 (2.4466, 3.8949) -> (2.4462, 3.8941)
  line L23 (2.4462, 3.8941) -> (1.9582, 3.1172)
  arc A12 (1.9582, 3.1172) -> (0.8196, 3.5889) centre (0, 0) ccw
  line L24 (0.8196, 3.5889) -> (1.0239, 4.4833)
  line L25 (1.0239, 4.4833) -> (1.024, 4.4841)
  spline S12 degree 5 poles (1.024, 4.4841) (1.0241, 4.4842) (1.0241, 4.4844) (1.0242, 4.4848) (1.0243, 4.4853) (1.0244, 4.486) (1.0246, 4.4869) (1.0248, 4.4879) (1.025, 4.489) (1.0252, 4.4903) (1.0254, 4.4916) (1.0257, 4.4931) (1.0259, 4.4947) (1.0262, 4.4963) (1.0264, 4.4981) (1.0267, 4.5) (1.027, 4.502) (1.0272, 4.5042) (1.0275, 4.5064) (1.0278, 4.5087) (1.0281, 4.5111) (1.0284, 4.5136) (1.0287, 4.5162) (1.0289, 4.5189) (1.0292, 4.5218) (1.0295, 4.5247) (1.0297, 4.5277) (1.03, 4.5308) (1.0302, 4.534) (1.0305, 4.5372) (1.0307, 4.5406) (1.0309, 4.5441) (1.0311, 4.5476) (1.0313, 4.5513) (1.0315, 4.555) (1.0317, 4.5588) (1.0319, 4.5627) (1.032, 4.5667) (1.0321, 4.5708) (1.0322, 4.575) (1.0323, 4.5792) (1.0324, 4.5835) (1.0325, 4.5879) (1.0325, 4.5924) (1.0325, 4.597) (1.0325, 4.6016) (1.0325, 4.6064) (1.0324, 4.6111) (1.0324, 4.616) (1.0323, 4.621) (1.0322, 4.626) (1.032, 4.6311) (1.0319, 4.6363) (1.0317, 4.6415) (1.0315, 4.6468) (1.0312, 4.6522) (1.031, 4.6577) (1.0307, 4.6632) (1.0303, 4.6688) (1.03, 4.6745) (1.0296, 4.6802) (1.0292, 4.686) (1.0288, 4.6919) (1.0283, 4.6978) (1.0278, 4.7038) (1.0272, 4.7099) (1.0267, 4.716) (1.0261, 4.7222) (1.0255, 4.7285) (1.0248, 4.7348) (1.0241, 4.7412) (1.0234, 4.7476) (1.0226, 4.7541) (1.0218, 4.7607) (1.021, 4.7673) (1.0201, 4.774) (1.0192, 4.7807) (1.0182, 4.7875) (1.0173, 4.7944) (1.0162, 4.8013) (1.0152, 4.8083) (1.0141, 4.8153) (1.013, 4.8224) (1.0118, 4.8295) (1.0106, 4.8367) (1.0093, 4.8439) (1.0081, 4.8512) (1.0067, 4.8585) (1.0054, 4.8659) (1.004, 4.8734) (1.0025, 4.8809) (1.001, 4.8884) (0.9995, 4.896) (0.9979, 4.9037) (0.9963, 4.9114) (0.9947, 4.9191) (0.993, 4.9269) (0.9912, 4.9347) (0.9894, 4.9426) (0.9876, 4.9505) (0.9858, 4.9585) (0.9838, 4.9665) (0.9819, 4.9746) (0.9799, 4.9827) (0.9778, 4.9908) (0.9757, 4.999) (0.9736, 5.0073) (0.9714, 5.0155) (0.9692, 5.0239) (0.9669, 5.0322) (0.9646, 5.0406) (0.9623, 5.0491) (0.9599, 5.0576) (0.9574, 5.0661) (0.9549, 5.0746) (0.9524, 5.0832) (0.9498, 5.0919) (0.9471, 5.1005) (0.9444, 5.1092) (0.9417, 5.118) (0.9389, 5.1268) (0.9361, 5.1356) (0.9332, 5.1444) (0.9303, 5.1533) (0.9273, 5.1623) (0.9243, 5.1712) (0.9212, 5.1802) (0.9181, 5.1892) (0.9149, 5.1983) (0.9117, 5.2074) (0.9084, 5.2165) (0.9051, 5.2256) (0.9017, 5.2348) (0.8983, 5.244) (0.8948, 5.2533) (0.8913, 5.2626) (0.8877, 5.2719) (0.8841, 5.2812) (0.8804, 5.2905) (0.8767, 5.2999) (0.8729, 5.3094) (0.8691, 5.3188) (0.8652, 5.3283) (0.8613, 5.3378) (0.8573, 5.3473) (0.8533, 5.3568) (0.8492, 5.3664) (0.8451, 5.376) (0.8409, 5.3856) (0.8367, 5.3953) (0.8324, 5.4049) (0.8281, 5.4146) (0.8237, 5.4244) (0.8192, 5.4341) (0.8147, 5.4439) (0.8102, 5.4537) (0.8056, 5.4635) (0.8009, 5.4733) (0.7962, 5.4831) (0.7915, 5.493) (0.7867, 5.5029) (0.7818, 5.5128) (0.7769, 5.5227) (0.7719, 5.5327) (0.7669, 5.5426) (0.7618, 5.5526) (0.7567, 5.5626) (0.7515, 5.5726) (0.7463, 5.5827) (0.741, 5.5927) (0.7356, 5.6028) (0.7302, 5.6129) (0.7248, 5.623) (0.7193, 5.6331) (0.7137, 5.6432) (0.7081, 5.6534) (0.7024, 5.6636) (0.6967, 5.6737) (0.6909, 5.6839) (0.6851, 5.6941) (0.6792, 5.7043) (0.6733, 5.7146) (0.6673, 5.7248) (0.6613, 5.7351) (0.6552, 5.7453) (0.649, 5.7556) (0.6428, 5.7659) (0.6365, 5.7762) (0.6302, 5.7865) (0.6239, 5.7968) (0.6174, 5.8071) (0.611, 5.8175) (0.6044, 5.8278) (0.5978, 5.8382) (0.5912, 5.8485) (0.5845, 5.8589) (0.5777, 5.8693) (0.5709, 5.8797) (0.5641, 5.8901) (0.5572, 5.9005) (0.5502, 5.9109) (0.5432, 5.9213) (0.5361, 5.9317) (0.529, 5.9421) (0.5218, 5.9525) (0.5145, 5.963) (0.5072, 5.9734) (0.4999, 5.9839) (0.4925, 5.9943) (0.485, 6.0048) (0.4775, 6.0152) (0.4699, 6.0257) (0.4623, 6.0361) (0.4546, 6.0466) (0.4469, 6.057) (0.4391, 6.0675) (0.4313, 6.078) (0.4234, 6.0884) (0.4154, 6.0989) (0.4074, 6.1094) (0.3993, 6.1199) (0.3912, 6.1303) (0.383, 6.1408) (0.3748, 6.1513) (0.3665, 6.1617) (0.3582, 6.1722) (0.3498, 6.1827) (0.3414, 6.1931) (0.3329, 6.2036) (0.3243, 6.2141) (0.3157, 6.2245) (0.3071, 6.235) (0.2983, 6.2454) (0.2896, 6.2559) (0.2807, 6.2663) (0.2719, 6.2768) (0.2629, 6.2872) (0.2539, 6.2976) (0.2449, 6.3081) (0.2358, 6.3185) (0.2267, 6.3289) (0.2193, 6.3372) (0.2137, 6.3435) (0.21, 6.3476) (0.2082, 6.3497) knots 0 0 0 0 0 0 0.00416667 0.00833333 0.0125 0.01666667 0.02083333 0.025 0.02916667 0.03333333 0.0375 0.04166667 0.04583333 0.05 0.05416667 0.05833333 0.0625 0.06666667 0.07083333 0.075 0.07916667 0.08333333 0.0875 0.09166667 0.09583333 0.1 0.10416667 0.10833333 0.1125 0.11666667 0.12083333 0.125 0.12916667 0.13333333 0.1375 0.14166667 0.14583333 0.15 0.15416667 0.15833333 0.1625 0.16666667 0.17083333 0.175 0.17916667 0.18333333 0.1875 0.19166667 0.19583333 0.2 0.20416667 0.20833333 0.2125 0.21666667 0.22083333 0.225 0.22916667 0.23333333 0.2375 0.24166667 0.24583333 0.25 0.25416667 0.25833333 0.2625 0.26666667 0.27083333 0.275 0.27916667 0.28333333 0.2875 0.29166667 0.29583333 0.3 0.30416667 0.30833333 0.3125 0.31666667 0.32083333 0.325 0.32916667 0.33333333 0.3375 0.34166667 0.34583333 0.35 0.35416667 0.35833333 0.3625 0.36666667 0.37083333 0.375 0.37916667 0.38333333 0.3875 0.39166667 0.39583333 0.4 0.40416667 0.40833333 0.4125 0.41666667 0.42083333 0.425 0.42916667 0.43333333 0.4375 0.44166667 0.44583333 0.45 0.45416667 0.45833333 0.4625 0.46666667 0.47083333 0.475 0.47916667 0.48333333 0.4875 0.49166667 0.49583333 0.5 0.50416667 0.50833333 0.5125 0.51666667 0.52083333 0.525 0.52916667 0.53333333 0.5375 0.54166667 0.54583333 0.55 0.55416667 0.55833333 0.5625 0.56666667 0.57083333 0.575 0.57916667 0.58333333 0.5875 0.59166667 0.59583333 0.6 0.60416667 0.60833333 0.6125 0.61666667 0.62083333 0.625 0.62916667 0.63333333 0.6375 0.64166667 0.64583333 0.65 0.65416667 0.65833333 0.6625 0.66666667 0.67083333 0.675 0.67916667 0.68333333 0.6875 0.69166667 0.69583333 0.7 0.70416667 0.70833333 0.7125 0.71666667 0.72083333 0.725 0.72916667 0.73333333 0.7375 0.74166667 0.74583333 0.75 0.75416667 0.75833333 0.7625 0.76666667 0.77083333 0.775 0.77916667 0.78333333 0.7875 0.79166667 0.79583333 0.8 0.80416667 0.80833333 0.8125 0.81666667 0.82083333 0.825 0.82916667 0.83333333 0.8375 0.84166667 0.84583333 0.85 0.85416667 0.85833333 0.8625 0.86666667 0.87083333 0.875 0.87916667 0.88333333 0.8875 0.89166667 0.89583333 0.9 0.90416667 0.90833333 0.9125 0.91666667 0.92083333 0.925 0.92916667 0.93333333 0.9375 0.94166667 0.94583333 0.95 0.95416667 0.95833333 0.9625 0.96666667 0.97083333 0.975 0.97916667 0.98333333 0.9875 0.99166667 0.99583333 1 1 1 1 1 1
  arc A13 (0.2082, 6.3497) -> (-0.2082, 6.3497) centre (0, 0) ccw
  spline S13 degree 5 poles (-0.2082, 6.3497) (-0.21, 6.3476) (-0.2137, 6.3435) (-0.2193, 6.3372) (-0.2267, 6.3289) (-0.2358, 6.3185) (-0.2449, 6.3081) (-0.2539, 6.2976) (-0.2629, 6.2872) (-0.2719, 6.2768) (-0.2807, 6.2663) (-0.2896, 6.2559) (-0.2983, 6.2454) (-0.3071, 6.235) (-0.3157, 6.2245) (-0.3243, 6.2141) (-0.3329, 6.2036) (-0.3414, 6.1931) (-0.3498, 6.1827) (-0.3582, 6.1722) (-0.3665, 6.1617) (-0.3748, 6.1513) (-0.383, 6.1408) (-0.3912, 6.1303) (-0.3993, 6.1199) (-0.4074, 6.1094) (-0.4154, 6.0989) (-0.4234, 6.0884) (-0.4313, 6.078) (-0.4391, 6.0675) (-0.4469, 6.057) (-0.4546, 6.0466) (-0.4623, 6.0361) (-0.4699, 6.0257) (-0.4775, 6.0152) (-0.485, 6.0048) (-0.4925, 5.9943) (-0.4999, 5.9839) (-0.5072, 5.9734) (-0.5145, 5.963) (-0.5218, 5.9525) (-0.529, 5.9421) (-0.5361, 5.9317) (-0.5432, 5.9213) (-0.5502, 5.9109) (-0.5572, 5.9005) (-0.5641, 5.8901) (-0.5709, 5.8797) (-0.5777, 5.8693) (-0.5845, 5.8589) (-0.5912, 5.8485) (-0.5978, 5.8382) (-0.6044, 5.8278) (-0.611, 5.8175) (-0.6174, 5.8071) (-0.6239, 5.7968) (-0.6302, 5.7865) (-0.6365, 5.7762) (-0.6428, 5.7659) (-0.649, 5.7556) (-0.6552, 5.7453) (-0.6613, 5.7351) (-0.6673, 5.7248) (-0.6733, 5.7146) (-0.6792, 5.7043) (-0.6851, 5.6941) (-0.6909, 5.6839) (-0.6967, 5.6737) (-0.7024, 5.6636) (-0.7081, 5.6534) (-0.7137, 5.6432) (-0.7193, 5.6331) (-0.7248, 5.623) (-0.7302, 5.6129) (-0.7356, 5.6028) (-0.741, 5.5927) (-0.7463, 5.5827) (-0.7515, 5.5726) (-0.7567, 5.5626) (-0.7618, 5.5526) (-0.7669, 5.5426) (-0.7719, 5.5327) (-0.7769, 5.5227) (-0.7818, 5.5128) (-0.7867, 5.5029) (-0.7915, 5.493) (-0.7962, 5.4831) (-0.8009, 5.4733) (-0.8056, 5.4635) (-0.8102, 5.4537) (-0.8147, 5.4439) (-0.8192, 5.4341) (-0.8237, 5.4244) (-0.8281, 5.4146) (-0.8324, 5.4049) (-0.8367, 5.3953) (-0.8409, 5.3856) (-0.8451, 5.376) (-0.8492, 5.3664) (-0.8533, 5.3568) (-0.8573, 5.3473) (-0.8613, 5.3378) (-0.8652, 5.3283) (-0.8691, 5.3188) (-0.8729, 5.3094) (-0.8767, 5.2999) (-0.8804, 5.2905) (-0.8841, 5.2812) (-0.8877, 5.2719) (-0.8913, 5.2626) (-0.8948, 5.2533) (-0.8983, 5.244) (-0.9017, 5.2348) (-0.9051, 5.2256) (-0.9084, 5.2165) (-0.9117, 5.2074) (-0.9149, 5.1983) (-0.9181, 5.1892) (-0.9212, 5.1802) (-0.9243, 5.1712) (-0.9273, 5.1623) (-0.9303, 5.1533) (-0.9332, 5.1444) (-0.9361, 5.1356) (-0.9389, 5.1268) (-0.9417, 5.118) (-0.9444, 5.1092) (-0.9471, 5.1005) (-0.9498, 5.0919) (-0.9524, 5.0832) (-0.9549, 5.0746) (-0.9574, 5.0661) (-0.9599, 5.0576) (-0.9623, 5.0491) (-0.9646, 5.0406) (-0.9669, 5.0322) (-0.9692, 5.0239) (-0.9714, 5.0155) (-0.9736, 5.0073) (-0.9757, 4.999) (-0.9778, 4.9908) (-0.9799, 4.9827) (-0.9819, 4.9746) (-0.9838, 4.9665) (-0.9858, 4.9585) (-0.9876, 4.9505) (-0.9894, 4.9426) (-0.9912, 4.9347) (-0.993, 4.9269) (-0.9947, 4.9191) (-0.9963, 4.9114) (-0.9979, 4.9037) (-0.9995, 4.896) (-1.001, 4.8884) (-1.0025, 4.8809) (-1.004, 4.8734) (-1.0054, 4.8659) (-1.0067, 4.8585) (-1.0081, 4.8512) (-1.0093, 4.8439) (-1.0106, 4.8367) (-1.0118, 4.8295) (-1.013, 4.8224) (-1.0141, 4.8153) (-1.0152, 4.8083) (-1.0162, 4.8013) (-1.0173, 4.7944) (-1.0182, 4.7875) (-1.0192, 4.7807) (-1.0201, 4.774) (-1.021, 4.7673) (-1.0218, 4.7607) (-1.0226, 4.7541) (-1.0234, 4.7476) (-1.0241, 4.7412) (-1.0248, 4.7348) (-1.0255, 4.7285) (-1.0261, 4.7222) (-1.0267, 4.716) (-1.0272, 4.7099) (-1.0278, 4.7038) (-1.0283, 4.6978) (-1.0288, 4.6919) (-1.0292, 4.686) (-1.0296, 4.6802) (-1.03, 4.6745) (-1.0303, 4.6688) (-1.0307, 4.6632) (-1.031, 4.6577) (-1.0312, 4.6522) (-1.0315, 4.6468) (-1.0317, 4.6415) (-1.0319, 4.6363) (-1.032, 4.6311) (-1.0322, 4.626) (-1.0323, 4.621) (-1.0324, 4.616) (-1.0324, 4.6111) (-1.0325, 4.6064) (-1.0325, 4.6016) (-1.0325, 4.597) (-1.0325, 4.5924) (-1.0325, 4.5879) (-1.0324, 4.5835) (-1.0323, 4.5792) (-1.0322, 4.575) (-1.0321, 4.5708) (-1.032, 4.5667) (-1.0319, 4.5627) (-1.0317, 4.5588) (-1.0315, 4.555) (-1.0313, 4.5513) (-1.0311, 4.5476) (-1.0309, 4.5441) (-1.0307, 4.5406) (-1.0305, 4.5372) (-1.0302, 4.534) (-1.03, 4.5308) (-1.0297, 4.5277) (-1.0295, 4.5247) (-1.0292, 4.5218) (-1.0289, 4.5189) (-1.0287, 4.5162) (-1.0284, 4.5136) (-1.0281, 4.5111) (-1.0278, 4.5087) (-1.0275, 4.5064) (-1.0272, 4.5042) (-1.027, 4.502) (-1.0267, 4.5) (-1.0264, 4.4981) (-1.0262, 4.4963) (-1.0259, 4.4947) (-1.0257, 4.4931) (-1.0254, 4.4916) (-1.0252, 4.4903) (-1.025, 4.489) (-1.0248, 4.4879) (-1.0246, 4.4869) (-1.0244, 4.486) (-1.0243, 4.4853) (-1.0242, 4.4848) (-1.0241, 4.4844) (-1.0241, 4.4842) (-1.024, 4.4841) knots -1 -1 -1 -1 -1 -1 -0.99583333 -0.99166667 -0.9875 -0.98333333 -0.97916667 -0.975 -0.97083333 -0.96666667 -0.9625 -0.95833333 -0.95416667 -0.95 -0.94583333 -0.94166667 -0.9375 -0.93333333 -0.92916667 -0.925 -0.92083333 -0.91666667 -0.9125 -0.90833333 -0.90416667 -0.9 -0.89583333 -0.89166667 -0.8875 -0.88333333 -0.87916667 -0.875 -0.87083333 -0.86666667 -0.8625 -0.85833333 -0.85416667 -0.85 -0.84583333 -0.84166667 -0.8375 -0.83333333 -0.82916667 -0.825 -0.82083333 -0.81666667 -0.8125 -0.80833333 -0.80416667 -0.8 -0.79583333 -0.79166667 -0.7875 -0.78333333 -0.77916667 -0.775 -0.77083333 -0.76666667 -0.7625 -0.75833333 -0.75416667 -0.75 -0.74583333 -0.74166667 -0.7375 -0.73333333 -0.72916667 -0.725 -0.72083333 -0.71666667 -0.7125 -0.70833333 -0.70416667 -0.7 -0.69583333 -0.69166667 -0.6875 -0.68333333 -0.67916667 -0.675 -0.67083333 -0.66666667 -0.6625 -0.65833333 -0.65416667 -0.65 -0.64583333 -0.64166667 -0.6375 -0.63333333 -0.62916667 -0.625 -0.62083333 -0.61666667 -0.6125 -0.60833333 -0.60416667 -0.6 -0.59583333 -0.59166667 -0.5875 -0.58333333 -0.57916667 -0.575 -0.57083333 -0.56666667 -0.5625 -0.55833333 -0.55416667 -0.55 -0.54583333 -0.54166667 -0.5375 -0.53333333 -0.52916667 -0.525 -0.52083333 -0.51666667 -0.5125 -0.50833333 -0.50416667 -0.5 -0.49583333 -0.49166667 -0.4875 -0.48333333 -0.47916667 -0.475 -0.47083333 -0.46666667 -0.4625 -0.45833333 -0.45416667 -0.45 -0.44583333 -0.44166667 -0.4375 -0.43333333 -0.42916667 -0.425 -0.42083333 -0.41666667 -0.4125 -0.40833333 -0.40416667 -0.4 -0.39583333 -0.39166667 -0.3875 -0.38333333 -0.37916667 -0.375 -0.37083333 -0.36666667 -0.3625 -0.35833333 -0.35416667 -0.35 -0.34583333 -0.34166667 -0.3375 -0.33333333 -0.32916667 -0.325 -0.32083333 -0.31666667 -0.3125 -0.30833333 -0.30416667 -0.3 -0.29583333 -0.29166667 -0.2875 -0.28333333 -0.27916667 -0.275 -0.27083333 -0.26666667 -0.2625 -0.25833333 -0.25416667 -0.25 -0.24583333 -0.24166667 -0.2375 -0.23333333 -0.22916667 -0.225 -0.22083333 -0.21666667 -0.2125 -0.20833333 -0.20416667 -0.2 -0.19583333 -0.19166667 -0.1875 -0.18333333 -0.17916667 -0.175 -0.17083333 -0.16666667 -0.1625 -0.15833333 -0.15416667 -0.15 -0.14583333 -0.14166667 -0.1375 -0.13333333 -0.12916667 -0.125 -0.12083333 -0.11666667 -0.1125 -0.10833333 -0.10416667 -0.1 -0.09583333 -0.09166667 -0.0875 -0.08333333 -0.07916667 -0.075 -0.07083333 -0.06666667 -0.0625 -0.05833333 -0.05416667 -0.05 -0.04583333 -0.04166667 -0.0375 -0.03333333 -0.02916667 -0.025 -0.02083333 -0.01666667 -0.0125 -0.00833333 -0.00416667 0 0 0 0 0 0
  line L26 (-1.024, 4.4841) -> (-1.0239, 4.4833)
  line L27 (-1.0239, 4.4833) -> (-0.8196, 3.5889)
  arc A14 (-0.8196, 3.5889) -> (-1.9582, 3.1172) centre (0, 0) ccw
  line L28 (-1.9582, 3.1172) -> (-2.4462, 3.8941)
  line L29 (-2.4462, 3.8941) -> (-2.4466, 3.8949)